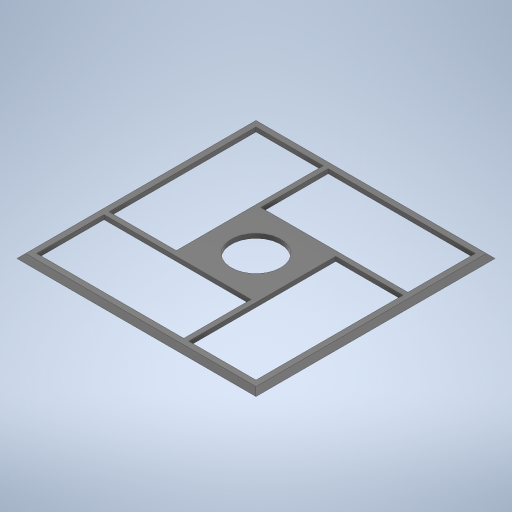
# Autodesk Inventor part: Lampara2base
Saved by Autodesk Inventor 2024 (Build 280153000, 153)
## iProperties
Created: 2023-12-01
Part Number: Lampara2base
Material: Genérico
Document SubType Name: Modeling
Designer: sergi
Density: 1 g/cm^3
Appearance: Valor por defecto
Author: sergi
Autodesk Inventor part; units mm, degrees
ref_plane "YZ Plane" through (0, 0, 0) normal (1, 0, 0) x (0, 1, 0)
ref_plane "XZ Plane" through (0, 0, 0) normal (0, 1, 0) x (-1, 0, 0)
ref_plane "XY Plane" through (0, 0, 0) normal (0, 0, 1) x (1, 0, 0)
sketch "Boceto1" plane through (0, 0, 0) normal (0, 1, 0) x (-1, 0, 0)
  line L0 (0, 0) -> (220.8, 0)
  line L1 (220.8, 0) -> (220.8, -220.8)
  line L2 (220.8, -220.8) -> (0, -220.8)
  line L3 (0, -220.8) -> (0, 0)
  line L4 (211.6, -211.6) -> (211.6, -147.2)
  line L5 (211.6, -9.2) -> (156.4, -9.2)
  line L6 (9.2, -211.6) -> (73.6, -211.6)
  line L7 (73.6, -211.6) -> (73.6, -209.3)
  line L8 (75.9, -71.3) -> (211.6, -71.3)
  line L9 (149.5, -211.6) -> (149.5, -75.9)
  line L10 (211.6, -9.2) -> (211.6, -71.3)
  line L11 (211.6, -75.9) -> (211.6, -82.8)
  line L12 (211.6, -211.6) -> (211.6, -75.9)
  line L13 (211.6, -71.3) -> (211.6, -9.2)
  line L14 (75.9, -75.9) -> (144.9, -75.9)
  line L15 (149.5, -75.9) -> (211.6, -75.9)
  line L16 (9.2, -149.5) -> (144.9, -149.5)
  line L17 (144.9, -211.6) -> (144.9, -149.5)
  line L18 (144.9, -144.9) -> (144.9, -75.9)
  line L19 (71.3, -144.9) -> (71.3, -9.2)
  line L20 (9.2, -144.9) -> (71.3, -144.9)
  line L21 (75.9, -144.9) -> (144.9, -144.9)
  line L22 (75.9, -144.9) -> (75.9, -75.9)
  line L23 (75.9, -71.3) -> (75.9, -9.2)
  line L24 (211.6, -9.2) -> (75.9, -9.2)
  line L25 (71.3, -9.2) -> (9.2, -9.2)
  line L26 (9.2, -9.2) -> (9.2, -144.9)
  line L27 (9.2, -149.5) -> (9.2, -211.6)
  line L28 (9.2, -211.6) -> (144.9, -211.6)
  line L29 (149.5, -211.6) -> (211.6, -211.6)
  dimension "d0" = 220.8
  dimension "d1" = 220.8
  constraints: 60 end point, 10 parallel, 5 perpendicular, 4 point on line, 1 horizontal
  measures "d0" distance of L1.end L2.end
  measures "d1" distance of L0.end L1.end
extrude "Extrusión1" add sketch "Boceto1" along normal blind 4
chamfer "Chaflán1" distance 4 angle 45 4 edges at (-220.8, 4, -110.4) (-110.4, 4, 0) (0, 4, -110.4) (-110.4, 4, -220.8) measured on face at (-121.9, 4, -217.7333)
sketch "Boceto2" plane through (0, 0, 0) normal (0, -1, 0) x (1, 0, 0)
  line L0 (-216.8, -4) -> (-216.8, -216.8) projected
  line L1 (0, -220.8) -> (-220.8, -220.8) projected
  line L2 (0, 0) -> (0, -220.8) projected
  line L3 (-220.8, 0) -> (0, 0) projected
  line L4 (-220.8, -220.8) -> (-220.8, 0) projected
  line L5 (-9.2, -211.6) -> (-9.2, -149.5) projected
  line L6 (-144.9, -211.6) -> (-9.2, -211.6) projected
  line L7 (-144.9, -149.5) -> (-144.9, -211.6) projected
  line L8 (-9.2, -149.5) -> (-144.9, -149.5) projected
  line L9 (-71.3, -144.9) -> (-9.2, -144.9) projected
  line L10 (-71.3, -9.2) -> (-71.3, -144.9) projected
  line L11 (-9.2, -9.2) -> (-71.3, -9.2) projected
  line L12 (-9.2, -144.9) -> (-9.2, -9.2) projected
  line L13 (-75.9, -144.9) -> (-75.9, -75.9) projected
  line L14 (-144.9, -144.9) -> (-75.9, -144.9) projected
  line L15 (-144.9, -75.9) -> (-144.9, -144.9) projected
  line L16 (-75.9, -75.9) -> (-144.9, -75.9) projected
  line L17 (-149.5, -75.9) -> (-211.6, -75.9) projected
  line L18 (-149.5, -211.6) -> (-149.5, -75.9) projected
  line L19 (-211.6, -211.6) -> (-149.5, -211.6) projected
  line L20 (-211.6, -75.9) -> (-211.6, -211.6) projected
  line L21 (-75.9, -71.3) -> (-75.9, -9.2) projected
  line L22 (-211.6, -71.3) -> (-75.9, -71.3) projected
  line L23 (-211.6, -9.2) -> (-211.6, -71.3) projected
  line L24 (-75.9, -9.2) -> (-211.6, -9.2) projected
  circle A0 centre (-110.4, -110.4) radius 34.5
  circle A1 centre (-110.4, -110.4) radius 22.8
  dimension "d31" = 45.6
  constraints: 3 tangent, 2 centre point, 1 coincident
  measures "d31" diameter of A1
extrude "Extrusión2" add sketch "Boceto2" against normal blind 4 contours L14 A0 L13 | A0 L16 L13 | A0 | L14 L15 A0 | A0 L15 L16
